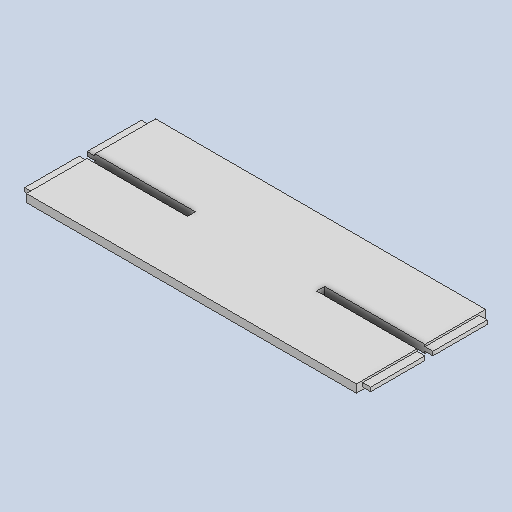
# Autodesk Inventor part: Sustainable Chair_V4 - Lateral Support
Saved by Autodesk Inventor 2025.2 (Build 292293000, 293)
## iProperties
Created: 2025-03-03
Part Number: Sustainable Chair_V4 - Lateral Support
Material: Foam Board - V3
Document SubType Name: Modeling
Designer: Dylan
Density: 0.151132 g/cm^3
Appearance: Default(1)
Mass: 10.8188 g
Surface Area: 345.339 cm^2
Volume: 71.5847 cm^3
Author: Dylan
Autodesk Inventor part; units mm, degrees
ref_plane "YZ Plane" through (0, 0, 0) normal (1, 0, 0) x (0, 1, 0)
ref_plane "XZ Plane" through (0, 0, 0) normal (0, 1, 0) x (-1, 0, 0)
ref_plane "XY Plane" through (0, 0, 0) normal (0, 0, 1) x (1, 0, 0)
sketch "Sketch1" plane through (0, 0, 0) normal (0, 1, 0) x (-1, 0, 0)
  line L0 (0, 0) -> (197.626, 0)
  line L1 (197.626, 0) -> (197.626, -77.381)
  line L2 (197.626, -77.381) -> (0, -77.381)
  line L3 (0, -77.381) -> (0, 0)
  dimension "d0" = 197.626
  dimension "d1" = 77.381
  constraints: 8 end point, 2 parallel, 1 horizontal, 1 perpendicular
  measures "d0" distance of L1.end L2.end
  measures "d1" distance of L0.end L1.end
extrude "Extrusion1" add sketch "Sketch1" along normal blind 4.763
sketch "Sketch2" plane through (0, 4.763, 0) normal (0, 1, 0) x (1, 0, 0)
  line L0 (0, 41.072) -> (0, 36.309)
  line L1 (0, 36.309) -> (-60.123, 36.309)
  line L2 (-60.123, 36.309) -> (-60.123, 41.072)
  line L3 (-60.123, 41.072) -> (0, 41.072)
  line L4 (-197.626, 41.072) -> (-197.626, 36.309)
  line L5 (-197.626, 36.309) -> (-137.503, 36.309)
  line L6 (-137.503, 36.309) -> (-137.503, 41.072)
  line L7 (-137.503, 41.072) -> (-197.626, 41.072)
  dimension "d6" = 4.763
  dimension "d7" = 60.123
  constraints: 16 end point, 1 horizontal, 1 perpendicular, 1 vertical
  measures "d6" distance of L0.start L0.end
  measures "d7" distance of L0.end L1.end
extrude "Extrusion2" cut sketch "Sketch2" against normal blind 22
sketch "Sketch3" plane through (0, 0, 0) normal (1, 0, 0) x (0, 0, -1)
  line L0 (36.309, 3.572) -> (3.806, 3.572)
  line L1 (3.806, 3.572) -> (3.806, 1.191)
  line L2 (3.806, 1.191) -> (36.309, 1.191)
  line L3 (36.309, 3.572) -> (36.309, 1.191)
  line L4 (41.072, 3.572) -> (73.575, 3.572)
  line L5 (73.575, 3.572) -> (73.575, 1.191)
  line L6 (73.575, 1.191) -> (41.072, 1.191)
  line L7 (41.072, 3.572) -> (41.072, 1.191)
  dimension "d12" = 32.503
  constraints: 16 end point, 1 perpendicular, 1 vertical
  measures "d12" distance of L0.start L0.end
extrude "Extrusion3" add sketch "Sketch3" along normal blind 4.763
ref_plane "Work Plane1" through (-98.813, 0, 0) normal (1, 0, 0) x (0, 0, -1)
mirror "Mirror1" about plane through (-98.813, 0, 0) normal (1, 0, 0) of "Extrusion3"
body "Solid1"
